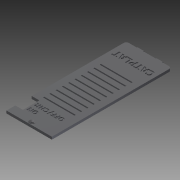
# Autodesk Inventor part: platform_top_cover_v2
Saved by Autodesk Inventor 2015 (Build 190159000, 159)
## iProperties
Created: 2016-05-02
Part Number: platform_top_cover_v2
Material: Plástico ABS
Document SubType Name: Modeling
Designer: JavierPC
Density: 1.06 g/cm^3
Appearance: Suave - Gris medio
Author: Javier Pérez de Frutos
Title: Cubierta
Autodesk Inventor part; units mm, degrees
ref_plane "YZ Plane" through (0, 0, 0) normal (1, 0, 0) x (0, 1, 0)
ref_plane "XZ Plane" through (0, 0, 0) normal (0, 1, 0) x (-1, 0, 0)
ref_plane "XY Plane" through (0, 0, 0) normal (0, 0, 1) x (1, 0, 0)
sketch "Boceto1" plane through (0, 0, 0) normal (0, 0, 1) x (1, 0, 0)
  line L0 (-16, 48.5) -> (16, 48.5)
  line L1 (18, 46.5) -> (18, -46.5)
  line L2 (18, -46.5) -> (-18, -46.5)
  line L3 (-18, -46.5) -> (-18, 46.5)
  line L4 (0, 14.9228) -> (0, -9.0046)
  line L5 (-13.5546, 0) -> (14.5, 0)
  arc A0 (18, 46.5) -> (16, 48.5) centre (16, 46.5) ccw
  arc A1 (-16, 48.5) -> (-18, 46.5) centre (-16, 46.5) ccw
  point P0 (0, 0)
  point P1 (18, 48.5)
  point P2 (0, 48.5)
  point P3 (-18, 0)
  dimension "d0" = 36
  dimension "d1" = 95
  dimension "d2" = 2
  constraints: 12 end point, 4 point on circle, 4 point on line, 4 tangent, 3 horizontal, 2 centre point, 2 midpoint, 2 parallel, 2 vertical, 1 equal radius, 1 perpendicular
  measures "d0" distance of L1.end L2.end
  measures "d1" distance of point (18, 48.5) L1.end
  measures "d2" radius of A0
extrude "Extrusión1" add sketch "Boceto1" along normal blind 2
sketch "Boceto2" plane through (-16, 48.5, 0) normal (0, 1, 0) x (1, 0, 0)
  line L0 (16, -6.6234) -> (16, 4.6993)
  line L1 (26, -1.5) -> (21, -1.5)
  line L2 (21, -1.5) -> (21, -0.5)
  line L3 (21, -0.5) -> (26, -0.5)
  line L4 (26, -0.5) -> (26, -1.5)
  line L5 (16, -0.962) -> (-3.465, -0.962)
  line L6 (6, -1.5) -> (11, -1.5)
  line L7 (11, -1.5) -> (11, -0.5)
  line L8 (11, -0.5) -> (6, -0.5)
  line L9 (6, -0.5) -> (6, -1.5)
  line L10 (32, -2) -> (0, -2) projected
  point P0 (16, 0)
  point P1 (11, -0.962)
  dimension "d7" = 5
  dimension "d8" = 1
  dimension "d9" = 10
  dimension "d35" = 0.5
  constraints: 20 end point, 4 symmetric about line, 3 horizontal, 2 parallel, 2 vertical, 1 midpoint, 1 perpendicular
  measures "d7" distance of L2.end L3.end
  measures "d8" distance of L1.end L2.end
  measures "d9" diameter of L2 L0
  measures "d35" distance between parallel lines of L10 L1
extrude "Extrusión2" add sketch "Boceto2" along normal blind 1.5
chamfer "Chaflán1" distance 0.5 angle 45 4 edges at (7.5, 50, 1.5) (7.5, 50, 0.5) (-7.5, 50, 1.5) (-7.5, 50, 0.5)
sketch "Boceto3" plane through (0, 0, 0) normal (0, 0, 1) x (1, 0, 0)
  line L0 (-12.5, -23) -> (12.5, -23)
  line L1 (12.5, -23) -> (12.5, -22)
  line L2 (12.5, -22) -> (-12.5, -22)
  line L3 (-12.5, -22) -> (-12.5, -23)
  line L4 (-25.7964, 0) -> (31.2947, 0)
  line L5 (0, 54.986) -> (0, -74.6304)
  line L6 (-12.5, -18) -> (12.5, -18)
  line L7 (12.5, -18) -> (12.5, -17)
  line L8 (12.5, -17) -> (-12.5, -17)
  line L9 (-12.5, -17) -> (-12.5, -18)
  line L10 (-12.5, -13) -> (12.5, -13)
  line L11 (12.5, -13) -> (12.5, -12)
  line L12 (12.5, -12) -> (-12.5, -12)
  line L13 (-12.5, -12) -> (-12.5, -13)
  line L14 (-12.5, -8) -> (12.5, -8)
  line L15 (12.5, -8) -> (12.5, -7)
  line L16 (12.5, -7) -> (-12.5, -7)
  line L17 (-12.5, -7) -> (-12.5, -8)
  line L18 (-12.5, -3) -> (12.5, -3)
  line L19 (12.5, -3) -> (12.5, -2)
  line L20 (12.5, -2) -> (-12.5, -2)
  line L21 (-12.5, -2) -> (-12.5, -3)
  line L22 (-12.5, 2) -> (12.5, 2)
  line L23 (12.5, 2) -> (12.5, 3)
  line L24 (12.5, 3) -> (-12.5, 3)
  line L25 (-12.5, 3) -> (-12.5, 2)
  line L26 (-12.5, 7) -> (12.5, 7)
  line L27 (12.5, 7) -> (12.5, 8)
  line L28 (12.5, 8) -> (-12.5, 8)
  line L29 (-12.5, 8) -> (-12.5, 7)
  line L30 (-12.5, 12) -> (12.5, 12)
  line L31 (12.5, 12) -> (12.5, 13)
  line L32 (12.5, 13) -> (-12.5, 13)
  line L33 (-12.5, 13) -> (-12.5, 12)
  line L34 (-12.5, 17) -> (12.5, 17)
  line L35 (12.5, 17) -> (12.5, 18)
  line L36 (12.5, 18) -> (-12.5, 18)
  line L37 (-12.5, 18) -> (-12.5, 17)
  line L38 (-12.5, 22) -> (12.5, 22)
  line L39 (12.5, 22) -> (12.5, 23)
  line L40 (12.5, 23) -> (-12.5, 23)
  line L41 (-12.5, 23) -> (-12.5, 22)
  line L42 (-12.5, 23) -> (-12.5, -23)
  point P0 (0, 0)
  point P1 (0, -23)
  point P2 (0, -18)
  point P3 (0, -13)
  point P4 (0, -8)
  point P5 (0, -3)
  point P6 (0, 2)
  point P7 (0, 7)
  point P8 (0, 12)
  point P9 (0, 17)
  point P10 (0, 22)
  point P11 (-12.5, 0)
  dimension "d15" = 25
  dimension "d16" = 1
  dimension "d19" = 5
  constraints: 86 end point, 3 horizontal, 3 vertical, 2 midpoint, 2 parallel, 2 perpendicular, 2 point on line, 81 other
  measures "d15" distance of L2.end L1.end
  measures "d16" distance of L1.end L0.end
  measures "d19" distance of L0.start L6.start
extrude "Extrusión3" cut sketch "Boceto3" along normal blind 2 contours L3 L2 L5 L0 | L5 L2 L1 L0 | L9 L8 L5 L6 | L5 L8 L7 L6 | L13 L12 L5 L10 | L5 L12 L11 L10 | L17 L16 L5 L14 | L5 L16 L15 L14 | L21 L20 L5 L18 | L5 L20 L19 L18 | L25 L24 L5 L22 | L5 L24 L23 L22 | L29 L28 L5 L26 | L5 L28 L27 L26 | L33 L32 L5 L30 | L5 L32 L31 L30 | L37 L36 L5 L34 | L5 L36 L35 L34 | L41 L40 L5 L38 | L5 L40 L39 L38
sketch "Boceto4" plane through (0, 0, 2) normal (0, 0, 1) x (1, 0, 0)
  line L0 (-18, -46.5) -> (18, -46.5)
  point P0 (0, 0)
  point P1 (0, -44)
  dimension "d26" = 2.5
  constraints: 2 end point
  measures "d26" distance from line of L0 point (0, -44)
hole "Agujero1" at (0, -44, 2) direction (0, 0, -1) diameter 2.4 end through all countersink diameter 4.6 countersink angle 90
sketch "Boceto5" plane through (0, 0, 0) normal (0, 0, 1) x (1, 0, 0)
  line L0 (-18, -46.5) -> (18, -46.5) projected
  line L1 (-18, -39.5) -> (-12, -39.5)
  line L2 (-12, -39.5) -> (-12, -26.5)
  line L3 (-12, -26.5) -> (-18, -26.5)
  line L4 (-18, -26.5) -> (-18, -39.5)
  point P0 (0, 0)
  dimension "d37" = 6
  dimension "d38" = 13
  dimension "d39" = 20
  constraints: 8 end point, 2 parallel, 1 horizontal, 1 perpendicular
  measures "d37" distance of L3.end L2.end
  measures "d38" distance of L2.end L1.end
  measures "d39" distance from line of L0 L3.end
extrude "Extrusión4" cut sketch "Boceto5" along normal blind 10
sketch "Boceto6" plane through (0, 0, 2) normal (0, 0, 1) x (1, 0, 0)
  line L0 (11.3581, -38.144) -> (-11.1055, -38.144) construction
  line L1 (-11.1055, -38.144) -> (-11.1055, -28.0475) construction
  line L2 (-11.1055, -28.0475) -> (11.3581, -28.0475) construction
  line L3 (11.3581, -28.0475) -> (11.3581, -38.144) construction
  line L4 (15.6176, 33.6222) -> (-15.3649, 33.6222) construction
  line L5 (-15.3649, 33.6222) -> (-15.3649, 39.2445) construction
  line L6 (-15.3649, 39.2445) -> (15.6176, 39.2445) construction
  line L7 (15.6176, 39.2445) -> (15.6176, 33.6222) construction
  line L8 (0.1263, -59.4886) -> (0.1263, 73.6506)
  spline S0 degree 2 poles (-7.2367, -36.3202) (-7.2367, -35.4693) (-6.3291, -34.4965) (-5.5406, -34.4965) knots 0 0 0 1 2 2 2
  spline S1 degree 2 poles (-5.5406, -34.4965) (-4.7493, -34.4965) (-3.8474, -35.4807) (-3.8474, -36.3202) knots 0 0 0 1 2 2 2
  spline S2 degree 2 poles (-3.8474, -36.3202) (-3.8474, -37.1626) (-4.7493, -38.144) (-5.5406, -38.144) knots 0 0 0 1 2 2 2
  spline S3 degree 2 poles (-5.5406, -38.144) (-6.3291, -38.144) (-7.2367, -37.1683) (-7.2367, -36.3202) knots 0 0 0 1 2 2 2
  spline S4 degree 2 poles (-6.3291, -36.3202) (-6.3291, -36.6351) (-6.2015, -37.0747) (-6.0909, -37.2137) knots 0 0 0 1 2 2 2
  spline S5 degree 2 poles (-6.0909, -37.2137) (-5.9803, -37.3583) (-5.6966, -37.4831) (-5.5435, -37.4831) knots 0 0 0 1 2 2 2
  spline S6 degree 2 poles (-5.5435, -37.4831) (-5.3818, -37.4831) (-5.118, -37.3668) (-4.9961, -37.2193) knots 0 0 0 1 2 2 2
  spline S7 degree 2 poles (-4.9961, -37.2193) (-4.8883, -37.0832) (-4.755, -36.6322) (-4.755, -36.3202) knots 0 0 0 1 2 2 2
  spline S8 degree 2 poles (-4.755, -36.3202) (-4.755, -35.9969) (-4.8826, -35.5715) (-4.9932, -35.4268) knots 0 0 0 1 2 2 2
  spline S9 degree 2 poles (-4.9932, -35.4268) (-5.1038, -35.2822) (-5.3903, -35.1574) (-5.5435, -35.1574) knots 0 0 0 1 2 2 2
  spline S10 degree 2 poles (-5.5435, -35.1574) (-5.6995, -35.1574) (-5.9888, -35.2907) (-6.0937, -35.4325) knots 0 0 0 1 2 2 2
  spline S11 degree 2 poles (-6.0937, -35.4325) (-6.2072, -35.5856) (-6.3291, -35.9912) (-6.3291, -36.3202) knots 0 0 0 1 2 2 2
  line L9 (-10.7566, -34.5702) -> (-9.9114, -34.5702)
  line L10 (-9.9114, -34.5702) -> (-8.5613, -37.0095)
  line L11 (-8.5613, -37.0095) -> (-8.5613, -34.5702)
  line L12 (-8.5613, -34.5702) -> (-7.7586, -34.5702)
  line L13 (-7.7586, -34.5702) -> (-7.7586, -38.0702)
  line L14 (-7.7586, -38.0702) -> (-8.8364, -38.0702)
  line L15 (-8.8364, -38.0702) -> (-9.9539, -36.065)
  line L16 (-9.9539, -36.065) -> (-9.9539, -38.0702)
  line L17 (-9.9539, -38.0702) -> (-10.7566, -38.0702)
  line L18 (-10.7566, -38.0702) -> (-10.7566, -34.5702)
  spline S12 degree 2 poles (7.8099, -30.5576) (7.8099, -29.7067) (8.7175, -28.7338) (9.506, -28.7338) knots 0 0 0 1 2 2 2
  spline S13 degree 2 poles (9.506, -28.7338) (10.2973, -28.7338) (11.1992, -29.718) (11.1992, -30.5576) knots 0 0 0 1 2 2 2
  spline S14 degree 2 poles (11.1992, -30.5576) (11.1992, -31.4) (10.2973, -32.3813) (9.506, -32.3813) knots 0 0 0 1 2 2 2
  spline S15 degree 2 poles (9.506, -32.3813) (8.7175, -32.3813) (7.8099, -31.4056) (7.8099, -30.5576) knots 0 0 0 1 2 2 2
  spline S16 degree 2 poles (8.7175, -30.5576) (8.7175, -30.8724) (8.8451, -31.312) (8.9557, -31.451) knots 0 0 0 1 2 2 2
  spline S17 degree 2 poles (8.9557, -31.451) (9.0663, -31.5957) (9.35, -31.7205) (9.5031, -31.7205) knots 0 0 0 1 2 2 2
  spline S18 degree 2 poles (9.5031, -31.7205) (9.6648, -31.7205) (9.9286, -31.6042) (10.0505, -31.4567) knots 0 0 0 1 2 2 2
  spline S19 degree 2 poles (10.0505, -31.4567) (10.1583, -31.3205) (10.2916, -30.8696) (10.2916, -30.5576) knots 0 0 0 1 2 2 2
  spline S20 degree 2 poles (10.2916, -30.5576) (10.2916, -30.2342) (10.164, -29.8088) (10.0534, -29.6641) knots 0 0 0 1 2 2 2
  spline S21 degree 2 poles (10.0534, -29.6641) (9.9428, -29.5195) (9.6563, -29.3947) (9.5031, -29.3947) knots 0 0 0 1 2 2 2
  spline S22 degree 2 poles (9.5031, -29.3947) (9.3471, -29.3947) (9.0578, -29.528) (8.9529, -29.6698) knots 0 0 0 1 2 2 2
  spline S23 degree 2 poles (8.9529, -29.6698) (8.8394, -29.823) (8.7175, -30.2286) (8.7175, -30.5576) knots 0 0 0 1 2 2 2
  line L19 (4.9452, -31.6411) -> (6.4144, -31.6411)
  line L20 (6.4144, -31.6411) -> (6.4144, -30.9802)
  line L21 (6.4144, -30.9802) -> (5.0615, -30.9802)
  line L22 (5.0615, -30.9802) -> (5.0615, -30.3137)
  line L23 (5.0615, -30.3137) -> (6.4144, -30.3137)
  line L24 (6.4144, -30.3137) -> (6.4144, -28.8076)
  line L25 (6.4144, -28.8076) -> (7.288, -28.8076)
  line L26 (7.288, -28.8076) -> (7.288, -32.3076)
  line L27 (7.288, -32.3076) -> (4.9452, -32.3076)
  line L28 (4.9452, -32.3076) -> (4.9452, -31.6411)
  line L29 (2.1486, -31.6411) -> (3.6178, -31.6411)
  line L30 (3.6178, -31.6411) -> (3.6178, -30.9802)
  line L31 (3.6178, -30.9802) -> (2.2649, -30.9802)
  line L32 (2.2649, -30.9802) -> (2.2649, -30.3137)
  line L33 (2.2649, -30.3137) -> (3.6178, -30.3137)
  line L34 (3.6178, -30.3137) -> (3.6178, -28.8076)
  line L35 (3.6178, -28.8076) -> (4.4914, -28.8076)
  line L36 (4.4914, -28.8076) -> (4.4914, -32.3076)
  line L37 (4.4914, -32.3076) -> (2.1486, -32.3076)
  line L38 (2.1486, -32.3076) -> (2.1486, -31.6411)
  line L39 (-0.2878, -32.4636) -> (1.1048, -28.0475)
  line L40 (1.1048, -28.0475) -> (1.7799, -28.0475)
  line L41 (1.7799, -28.0475) -> (0.3901, -32.4636)
  line L42 (0.3901, -32.4636) -> (-0.2878, -32.4636)
  spline S24 degree 2 poles (-2.5909, -28.7395) (-1.8024, -28.7395) (-0.8777, -29.6925) (-0.8777, -30.5547) knots 0 0 0 1 2 2 2
  spline S25 degree 2 poles (-0.8777, -30.5547) (-0.8777, -31.3858) (-1.8052, -32.3757) (-2.5937, -32.3757) knots 0 0 0 1 2 2 2
  spline S26 degree 2 poles (-2.5937, -32.3757) (-2.8008, -32.3757) (-3.1354, -32.3274) (-3.2886, -32.2877) knots 0 0 0 1 2 2 2
  spline S27 degree 2 poles (-3.2886, -32.2877) (-3.4077, -32.2509) (-3.6885, -32.1289) (-3.7764, -32.0835) knots 0 0 0 1 2 2 2
  line L43 (-3.7764, -32.0835) -> (-3.7764, -31.2496)
  line L44 (-3.7764, -31.2496) -> (-3.6885, -31.2496)
  spline S28 degree 2 poles (-3.6885, -31.2496) (-3.6233, -31.3064) (-3.4304, -31.4652) (-3.3085, -31.5389) knots 0 0 0 1 2 2 2
  spline S29 degree 2 poles (-3.3085, -31.5389) (-3.1865, -31.6155) (-2.8944, -31.7205) (-2.7327, -31.7205) knots 0 0 0 1 2 2 2
  spline S30 degree 2 poles (-2.7327, -31.7205) (-2.5427, -31.7205) (-2.2278, -31.6013) (-2.0832, -31.451) knots 0 0 0 1 2 2 2
  spline S31 degree 2 poles (-2.0832, -31.451) (-1.9527, -31.3177) (-1.7854, -30.8611) (-1.7854, -30.5519) knots 0 0 0 1 2 2 2
  spline S32 degree 2 poles (-1.7854, -30.5519) (-1.7854, -30.2257) (-1.9584, -29.7804) (-2.1002, -29.6443) knots 0 0 0 1 2 2 2
  spline S33 degree 2 poles (-2.1002, -29.6443) (-2.2363, -29.511) (-2.571, -29.3947) (-2.7384, -29.3947) knots 0 0 0 1 2 2 2
  spline S34 degree 2 poles (-2.7384, -29.3947) (-2.9114, -29.3947) (-3.2262, -29.511) (-3.334, -29.5819) knots 0 0 0 1 2 2 2
  spline S35 degree 2 poles (-3.334, -29.5819) (-3.4531, -29.6528) (-3.6318, -29.8031) (-3.697, -29.8627) knots 0 0 0 1 2 2 2
  line L45 (-3.697, -29.8627) -> (-3.7764, -29.8627)
  line L46 (-3.7764, -29.8627) -> (-3.7764, -29.0402)
  spline S36 degree 2 poles (-3.7764, -29.0402) (-3.68, -28.9948) (-3.4276, -28.8813) (-3.2914, -28.8416) knots 0 0 0 1 2 2 2
  spline S37 degree 2 poles (-3.2914, -28.8416) (-3.1269, -28.7906) (-2.8405, -28.7395) (-2.5909, -28.7395) knots 0 0 0 1 2 2 2
  line L47 (-7.2481, -28.8076) -> (-6.3688, -28.8076)
  line L48 (-6.3688, -28.8076) -> (-6.3688, -30.359)
  line L49 (-6.3688, -30.359) -> (-5.1747, -30.359)
  line L50 (-5.1747, -30.359) -> (-5.1747, -28.8076)
  line L51 (-5.1747, -28.8076) -> (-4.2955, -28.8076)
  line L52 (-4.2955, -28.8076) -> (-4.2955, -32.3076)
  line L53 (-4.2955, -32.3076) -> (-5.1747, -32.3076)
  line L54 (-5.1747, -32.3076) -> (-5.1747, -31.0256)
  line L55 (-5.1747, -31.0256) -> (-6.3688, -31.0256)
  line L56 (-6.3688, -31.0256) -> (-6.3688, -32.3076)
  line L57 (-6.3688, -32.3076) -> (-7.2481, -32.3076)
  line L58 (-7.2481, -32.3076) -> (-7.2481, -28.8076)
  line L59 (-11.2076, -28.8076) -> (-10.1383, -28.8076)
  line L60 (-10.1383, -28.8076) -> (-9.1654, -30.0924)
  line L61 (-9.1654, -30.0924) -> (-8.8478, -30.0924)
  line L62 (-8.8478, -30.0924) -> (-8.8478, -28.8076)
  line L63 (-8.8478, -28.8076) -> (-7.9742, -28.8076)
  line L64 (-7.9742, -28.8076) -> (-7.9742, -32.3076)
  line L65 (-7.9742, -32.3076) -> (-9.381, -32.3076)
  spline S38 degree 2 poles (-9.381, -32.3076) (-9.6731, -32.3076) (-10.1042, -32.2338) (-10.2886, -32.1204) knots 0 0 0 1 2 2 2
  spline S39 degree 2 poles (-10.2886, -32.1204) (-10.4758, -32.0013) (-10.697, -31.6297) (-10.697, -31.3461) knots 0 0 0 1 2 2 2
  spline S40 degree 2 poles (-10.697, -31.3461) (-10.697, -30.9462) (-10.334, -30.4441) (-10.0305, -30.2966) knots 0 0 0 1 2 2 2
  line L66 (-10.0305, -30.2966) -> (-11.2076, -28.8076)
  spline S41 degree 2 poles (-9.7951, -31.2355) (-9.7951, -31.3688) (-9.693, -31.5588) (-9.5767, -31.6099) knots 0 0 0 1 2 2 2
  spline S42 degree 2 poles (-9.5767, -31.6099) (-9.4944, -31.6439) (-9.2931, -31.6637) (-9.1427, -31.6637) knots 0 0 0 1 2 2 2
  line L67 (-9.1427, -31.6637) -> (-8.8478, -31.6637)
  line L68 (-8.8478, -31.6637) -> (-8.8478, -30.7221)
  line L69 (-8.8478, -30.7221) -> (-9.1002, -30.7221)
  spline S43 degree 2 poles (-9.1002, -30.7221) (-9.2817, -30.7221) (-9.5398, -30.7675) (-9.6277, -30.8384) knots 0 0 0 1 2 2 2
  spline S44 degree 2 poles (-9.6277, -30.8384) (-9.7128, -30.9064) (-9.7951, -31.088) (-9.7951, -31.2355) knots 0 0 0 1 2 2 2
  spline S45 degree 2 poles (12.9433, 38.8167) (14.0697, 38.8167) (15.3906, 37.4552) (15.3906, 36.2235) knots 0 0 0 1 2 2 2
  spline S46 degree 2 poles (15.3906, 36.2235) (15.3906, 35.0363) (14.0657, 33.6222) (12.9393, 33.6222) knots 0 0 0 1 2 2 2
  spline S47 degree 2 poles (12.9393, 33.6222) (12.6435, 33.6222) (12.1654, 33.6911) (11.9466, 33.7478) knots 0 0 0 1 2 2 2
  spline S48 degree 2 poles (11.9466, 33.7478) (11.7764, 33.8005) (11.3753, 33.9747) (11.2496, 34.0395) knots 0 0 0 1 2 2 2
  line L70 (11.2496, 34.0395) -> (11.2496, 35.2308)
  line L71 (11.2496, 35.2308) -> (11.3753, 35.2308)
  spline S49 degree 2 poles (11.3753, 35.2308) (11.4684, 35.1497) (11.744, 34.9228) (11.9182, 34.8175) knots 0 0 0 1 2 2 2
  spline S50 degree 2 poles (11.9182, 34.8175) (12.0924, 34.7081) (12.5098, 34.5581) (12.7407, 34.5581) knots 0 0 0 1 2 2 2
  spline S51 degree 2 poles (12.7407, 34.5581) (13.0122, 34.5581) (13.462, 34.7283) (13.6686, 34.9431) knots 0 0 0 1 2 2 2
  spline S52 degree 2 poles (13.6686, 34.9431) (13.855, 35.1335) (14.0941, 35.7859) (14.0941, 36.2275) knots 0 0 0 1 2 2 2
  spline S53 degree 2 poles (14.0941, 36.2275) (14.0941, 36.6935) (13.8469, 37.3296) (13.6443, 37.5241) knots 0 0 0 1 2 2 2
  spline S54 degree 2 poles (13.6443, 37.5241) (13.4498, 37.7146) (12.9717, 37.8807) (12.7326, 37.8807) knots 0 0 0 1 2 2 2
  spline S55 degree 2 poles (12.7326, 37.8807) (12.4855, 37.8807) (12.0357, 37.7146) (11.8817, 37.6133) knots 0 0 0 1 2 2 2
  spline S56 degree 2 poles (11.8817, 37.6133) (11.7116, 37.512) (11.4563, 37.2972) (11.3631, 37.2121) knots 0 0 0 1 2 2 2
  line L72 (11.3631, 37.2121) -> (11.2496, 37.2121)
  line L73 (11.2496, 37.2121) -> (11.2496, 38.3872)
  spline S57 degree 2 poles (11.2496, 38.3872) (11.3874, 38.452) (11.748, 38.6141) (11.9425, 38.6708) knots 0 0 0 1 2 2 2
  spline S58 degree 2 poles (11.9425, 38.6708) (12.1775, 38.7437) (12.5868, 38.8167) (12.9433, 38.8167) knots 0 0 0 1 2 2 2
  line L74 (11.0471, 38.7194) -> (9.3574, 33.7194)
  line L75 (9.3574, 33.7194) -> (7.9879, 33.7194)
  line L76 (7.9879, 33.7194) -> (6.2983, 38.7194)
  line L77 (6.2983, 38.7194) -> (7.5908, 38.7194)
  line L78 (7.5908, 38.7194) -> (7.9028, 37.6983)
  line L79 (7.9028, 37.6983) -> (9.4749, 37.6983)
  line L80 (9.4749, 37.6983) -> (9.791, 38.7194)
  line L81 (9.791, 38.7194) -> (11.0471, 38.7194)
  line L82 (8.1783, 36.7907) -> (8.6889, 35.1376)
  line L83 (8.6889, 35.1376) -> (9.2035, 36.7907)
  line L84 (9.2035, 36.7907) -> (8.1783, 36.7907)
  line L85 (4.8396, 38.7194) -> (4.8396, 34.6716)
  line L86 (4.8396, 34.6716) -> (6.3185, 34.6716)
  line L87 (6.3185, 34.6716) -> (6.3185, 33.7194)
  line L88 (6.3185, 33.7194) -> (2.1046, 33.7194)
  line L89 (2.1046, 33.7194) -> (2.1046, 34.6716)
  line L90 (2.1046, 34.6716) -> (3.5835, 34.6716)
  line L91 (3.5835, 34.6716) -> (3.5835, 38.7194)
  line L92 (3.5835, 38.7194) -> (4.8396, 38.7194)
  spline S59 degree 2 poles (-2.2552, 35.2956) (-2.2552, 35.644) (-2.0324, 36.2761) (-1.8257, 36.4868) knots 0 0 0 1 2 2 2
  spline S60 degree 2 poles (-1.8257, 36.4868) (-1.7001, 36.6205) (-1.3922, 36.8393) (-1.2098, 36.9163) knots 0 0 0 1 2 2 2
  spline S61 degree 2 poles (-1.2098, 36.9163) (-1.0235, 36.9933) (-0.5899, 37.0825) (-0.3225, 37.0825) knots 0 0 0 1 2 2 2
  line L93 (-0.3225, 37.0825) -> (0.3339, 37.0825)
  line L94 (0.3339, 37.0825) -> (0.3339, 38.7194)
  line L95 (0.3339, 38.7194) -> (1.59, 38.7194)
  line L96 (1.59, 38.7194) -> (1.59, 33.7194)
  line L97 (1.59, 33.7194) -> (-0.3508, 33.7194)
  spline S62 degree 2 poles (-0.3508, 33.7194) (-0.7803, 33.7194) (-1.4084, 33.8774) (-1.6636, 34.0476) knots 0 0 0 1 2 2 2
  spline S63 degree 2 poles (-1.6636, 34.0476) (-1.9473, 34.2381) (-2.2552, 34.862) (-2.2552, 35.2956) knots 0 0 0 1 2 2 2
  spline S64 degree 2 poles (-0.9667, 35.328) (-0.9667, 35.1133) (-0.7641, 34.8094) (-0.6264, 34.7526) knots 0 0 0 1 2 2 2
  spline S65 degree 2 poles (-0.6264, 34.7526) (-0.4481, 34.6757) (-0.1239, 34.6513) (0.1556, 34.6513) knots 0 0 0 1 2 2 2
  line L98 (0.1556, 34.6513) -> (0.3339, 34.6513)
  line L99 (0.3339, 34.6513) -> (0.3339, 36.1505)
  line L100 (0.3339, 36.1505) -> (0.2448, 36.1505)
  spline S66 degree 2 poles (0.2448, 36.1505) (0.0706, 36.1505) (-0.2455, 36.1424) (-0.363, 36.1222) knots 0 0 0 1 2 2 2
  spline S67 degree 2 poles (-0.363, 36.1222) (-0.4643, 36.106) (-0.6871, 36.0087) (-0.7479, 35.9479) knots 0 0 0 1 2 2 2
  spline S68 degree 2 poles (-0.7479, 35.9479) (-0.8776, 35.8264) (-0.9667, 35.5549) (-0.9667, 35.328) knots 0 0 0 1 2 2 2
  line L101 (-6.2625, 38.7194) -> (-2.9278, 38.7194)
  line L102 (-2.9278, 38.7194) -> (-2.9278, 33.7194)
  line L103 (-2.9278, 33.7194) -> (-4.1839, 33.7194)
  line L104 (-4.1839, 33.7194) -> (-4.1839, 37.7672)
  line L105 (-4.1839, 37.7672) -> (-6.2625, 37.7672)
  line L106 (-6.2625, 37.7672) -> (-6.2625, 38.7194)
  line L107 (-6.3233, 38.7194) -> (-8.0129, 33.7194)
  line L108 (-8.0129, 33.7194) -> (-9.3824, 33.7194)
  line L109 (-9.3824, 33.7194) -> (-11.0721, 38.7194)
  line L110 (-11.0721, 38.7194) -> (-9.7795, 38.7194)
  line L111 (-9.7795, 38.7194) -> (-9.4675, 37.6983)
  line L112 (-9.4675, 37.6983) -> (-7.8954, 37.6983)
  line L113 (-7.8954, 37.6983) -> (-7.5794, 38.7194)
  line L114 (-7.5794, 38.7194) -> (-6.3233, 38.7194)
  line L115 (-9.192, 36.7907) -> (-8.6815, 35.1376)
  line L116 (-8.6815, 35.1376) -> (-8.1669, 36.7907)
  line L117 (-8.1669, 36.7907) -> (-9.192, 36.7907)
  line L118 (-12.5307, 38.7194) -> (-12.5307, 34.6716)
  line L119 (-12.5307, 34.6716) -> (-11.0518, 34.6716)
  line L120 (-11.0518, 34.6716) -> (-11.0518, 33.7194)
  line L121 (-11.0518, 33.7194) -> (-15.2658, 33.7194)
  line L122 (-15.2658, 33.7194) -> (-15.2658, 34.6716)
  line L123 (-15.2658, 34.6716) -> (-13.7868, 34.6716)
  line L124 (-13.7868, 34.6716) -> (-13.7868, 38.7194)
  line L125 (-13.7868, 38.7194) -> (-12.5307, 38.7194)
  point P0 (0, 0)
  point P1 (0.1263, 33.6222)
  constraints: 2 end point, 2 vertical, 1 midpoint, 1 point on line, 4 other
extrude "Extrusión5" cut sketch "Boceto6" against normal blind 0.8 contours L42 L39 L8 | L8 L39 L40 L41 L42 | L97 S62 S63 S59 S60 S61 L93 L8 S66 S67 S68 S64 S65 | L8 S65 L98 L99 L100 S66 L93 L94 L95 L96 L97 | S0 S1 S2 S3 | L9 L10 L11 L12 L13 L14 L15 L16 L17 L18 | S12 S13 S14 S15 | L19 L20 L21 L22 L23 L24 L25 L26 L27 L28 | L29 L30 L31 L32 L33 L34 L35 L36 L37 L38 | S24 S25 S26 S27 L43 L44 S28 S29 S30 S31 S32 S33 S34 S35 L45 L46 S36 S37 | L47 L48 L49 L50 L51 L52 L53 L54 L55 L56 L57 L58 | L59 L60 L61 L62 L63 L64 L65 S38 S39 S40 L66 | S45 S46 S47 S48 L70 L71 S49 S50 S51 S52 S53 S54 S55 S56 L72 L73 S57 S58 | L74 L75 L76 L77 L78 L79 L80 L81 | L85 L86 L87 L88 L89 L90 L91 L92 | L101 L102 L103 L104 L105 L106 | L107 L108 L109 L110 L111 L112 L113 L114 | L118 L119 L120 L121 L122 L123 L124 L125
